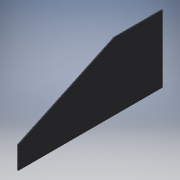
# Autodesk Inventor part: side
Saved by Autodesk Inventor 2018.1 (Build 221171000, 171)
## iProperties
Created: 2017-10-18
Part Number: side
Material: CFRP
Document SubType Name: Modeling
Designer: kuwano
Density: 1.43 g/cm^3
Appearance: カーボンファイバー
Mass: 270.201 g
Surface Area: 1293.01 cm^2
Volume: 188.951 cm^3
Author: kuwano
Autodesk Inventor part; units mm, degrees
ref_plane "YZ Plane" through (0, 0, 0) normal (1, 0, 0) x (0, 1, 0)
ref_plane "XZ Plane" through (0, 0, 0) normal (0, 1, 0) x (-1, 0, 0)
ref_plane "XY Plane" through (0, 0, 0) normal (0, 0, 1) x (1, 0, 0)
sketch "スケッチ1" plane through (0, 0, 0) normal (1, 0, 0) x (0, 1, 0)
  line L0 (105, -75.231) -> (-35, 225)
  line L1 (-35, 225) -> (-105, 225)
  line L2 (-105, 225) -> (-105, -225)
  line L3 (-105, -225) -> (105, -225)
  line L4 (105, -225) -> (105, -75.231)
  line L5 (-147, 0) -> (147, 0) projected
  line L6 (0, -315) -> (0, 315) projected
  point P0 (0, 0)
  point P1 (-105, 0)
  point P2 (0, -225)
  dimension "d0" = 70
  dimension "d1" = 450
  dimension "d2" = 210
  dimension "d3" = 25
  constraints: 10 end point, 3 perpendicular, 2 midpoint, 2 point on line, 1 horizontal
  measures "d0" distance of L0.end L1.end
  measures "d1" distance of L1.end L2.end
  measures "d2" distance of L2.end L3.end
  measures "d3" angle of L2 L0
extrude "押し出し1" add sketch "スケッチ1" along normal blind 3
